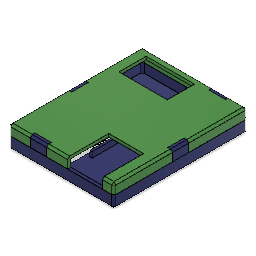
simple-case (Autodesk Fusion 360 design; units mm, degrees)
Autodesk Fusion 360 part; units mm, degrees
sketch "Sketch1" plane through (0, 0, 0) normal (0, 1, 0) x (1, 0, 0) in component "Giraffe"
  line L0 (-22.625, 29.5) -> (22.625, 29.5)
  line L1 (22.625, 29.5) -> (22.625, -29.5)
  line L2 (22.625, -29.5) -> (-22.625, -29.5)
  line L3 (-22.625, -29.5) -> (-22.625, 29.5)
  line L4 (-22.625, 29.5) -> (22.625, -29.5) construction
  line L5 (22.625, 29.5) -> (-22.625, -29.5) construction
  dimension "d1" = 59
  dimension "d2" = 45.25
extrude "Extrude1" add sketch "Sketch1" along normal blind 1.7 makes body 1 in component "Giraffe"
sketch "Sketch2" plane through (0, 0, 0) normal (0, -1, 0) x (1, 0, 0) in component "Giraffe"
  line L0 (22.625, 29.5) -> (-22.625, 29.5)
  line L1 (-22.625, 29.5) -> (-22.625, -29.5)
  line L2 (-22.625, -29.5) -> (22.625, -29.5)
  line L3 (22.625, -29.5) -> (22.625, 29.5)
  line L4 (-3.125, -12) -> (-3.125, 27)
  line L5 (-3.125, 27) -> (-18.125, 23)
  line L6 (-18.125, 23) -> (-18.125, -8)
  line L7 (-18.125, -8) -> (-3.125, -12)
  line L8 (-3.125, 7.5) -> (-13.2165, 7.5) construction
  dimension "d5" = 15
  dimension "d6" = 39
  dimension "d7" = 31
  dimension "d8" = 4.5
  dimension "d9" = 2.5
  measures "d5" distance of L4 L6
  measures "d8" distance of L1 L6
extrude "Extrude2" add sketch "Sketch2" along normal blind 15 separate body contours L4 L5 L6 L7 makes body 2 in component "Giraffe"
fillet "Fillet1" radius 3 4 edges at (-18.125, -7.5, 23) (-3.125, -7.5, 27) (-18.125, -7.5, -8) (-3.125, -7.5, -12) on bodies 2 in component "Giraffe"
sketch "Sketch3" plane through (0, 1.7, 0) normal (0, 1, 0) x (-1, 0, 0) in component "Giraffe"
  line L0 (22.625, 29.5) -> (-22.625, 29.5)
  line L1 (-22.625, 29.5) -> (-22.625, -29.5)
  line L2 (-22.625, -29.5) -> (22.625, -29.5)
  line L3 (22.625, -29.5) -> (22.625, 29.5)
  line L4 (-3.125, 12.5) -> (-20.125, 12.5)
  line L5 (-20.125, 12.5) -> (-20.125, 34.5)
  line L6 (-20.125, 34.5) -> (-3.125, 34.5)
  line L7 (-3.125, 34.5) -> (-3.125, 12.5)
  line L8 (20.325, -29.2) -> (-3.175, -29.2)
  line L9 (-3.175, -29.2) -> (-3.175, -15.95)
  line L10 (-3.175, -15.95) -> (20.325, -15.95)
  line L11 (20.325, -15.95) -> (20.325, -29.2)
  dimension "d13" = 13.25
  dimension "d14" = 23.5
  dimension "d15" = 0.3
  dimension "d16" = 2.3
  dimension "d17" = 17
  dimension "d18" = 22
  dimension "d19" = 2.5
  dimension "d20" = 17
  measures "d14" distance of origin
  measures "d15" distance of L2 L8
  measures "d16" distance of L3 L11
  measures "d18" distance of origin
  measures "d19" distance of L1 L5
  measures "d20" distance of L0 L4
extrude "Extrude4" add sketch "Sketch3" along normal blind 16 separate body contours L8 L9 L10 L11 makes body 3 in component "Giraffe"
extrude "Extrude3" add sketch "Sketch3" along normal blind 14 separate body contours L0 L4 L5 L7 | L0 L5 L6 L7 makes body 4 in component "Giraffe"
sketch "Sketch1 (2)" plane through (0, 1.7, 0) normal (0, 1, 0) x (-1, 0, 0) in component "Top"
  line L0 (22.625, 29.5) -> (-22.625, 29.5)
  line L1 (-22.625, 29.5) -> (-22.625, -29.5)
  line L2 (-22.625, -29.5) -> (22.625, -29.5)
  line L3 (22.625, -29.5) -> (22.625, 29.5)
  line L4 (-25.625, -32.5) -> (25.625, -32.5)
  line L5 (25.625, -32.5) -> (25.625, 32.5)
  line L6 (25.625, 32.5) -> (-25.625, 32.5)
  line L7 (-25.625, 32.5) -> (-25.625, -32.5)
  line L8 (-25.625, -32.5) -> (25.625, 32.5) construction
  line L9 (25.625, -32.5) -> (-25.625, 32.5) construction
  dimension "d25" = 3
  dimension "d26" = 3
  measures "d25" distance of L1 L7
  measures "d26" distance of L2 L4
extrude "Extrude1'" add sketch "Sketch1 (2)" along normal blind 5 separate body contours L0 L1 L2 L3 | L4 L5 L6 L7 makes body 5 in component "Top"
shell "Shell2" thickness 1.5 removed faces 1 at (8.5417, 1.7, 10.8333) on bodies 5 in component "Top"
combine "Combine1" operation cut target body 5 tool bodies 3 4 keep tools in component "Top"
sketch "Sketch2 (2)" plane through (0, 1.7, 0) normal (0, -1, 0) x (1, 0, 0) in component "Base"
  line L0 (3.125, 31) -> (3.125, 32.5)
  line L1 (3.125, 32.5) -> (-25.625, 32.5)
  line L2 (-25.625, 32.5) -> (-25.625, -32.5)
  line L3 (-25.625, -32.5) -> (25.625, -32.5)
  line L4 (25.625, -32.5) -> (25.625, 32.5)
  line L5 (25.625, 32.5) -> (20.125, 32.5)
  line L6 (20.125, 32.5) -> (20.125, 31)
  line L7 (20.125, 31) -> (24.125, 31)
  line L8 (24.125, 31) -> (24.125, -31)
  line L9 (24.125, -31) -> (-24.125, -31)
  line L10 (-24.125, -31) -> (-24.125, 31)
  line L11 (-24.125, 31) -> (3.125, 31)
  line L12 (25.625, -32.5) -> (-25.625, -32.5)
  line L13 (-25.625, -32.5) -> (-25.625, 32.5)
  line L14 (-25.625, 32.5) -> (25.625, 32.5)
  line L15 (25.625, 32.5) -> (25.625, -32.5)
extrude "Extrude1''" add sketch "Sketch2 (2)" along normal blind 6 separate body makes body 6 in component "Base"
shell "Shell1" thickness 1.5 removed faces 1 at (1.0417, 1.7, -10.8333) on bodies 6 in component "Base"
combine "Combine1'" operation cut target body 6 tool bodies 2 keep tools in component "Base"
sketch "Sketch3 (2)" plane through (0, 0, 0) normal (0, 0, 1) x (1, 0, 0) in component "Base"
  line L0 (25.625, 1.7) -> (24.125, 1.7)
  line L1 (24.125, 1.7) -> (24.125, 6.7)
  line L2 (24.125, 6.7) -> (25.625, 6.7)
  line L3 (25.625, 6.7) -> (25.625, 1.7)
  line L4 (25.625, 6.7) -> (-25.625, 6.7)
  line L5 (24.125, 5.2) -> (22.625, 6.7)
  line L6 (23.375, 5.95) -> (23.375, 6.7)
  dimension "d36" = 45
  dimension "d37" = 1.5
  measures "d36" angle of L1 L5
  measures "d37" distance of L4
extrude "Extrude2'" add sketch "Sketch3 (2)" along normal mid plane 8 separate body contours L0 L1 L2 L3 L4 | L1 L4 L5 L6 makes body 7 in component "Base"
chamfer "Chamfer1" distance 1 angle 45 1 edges at (25.625, 6.7, 0) on bodies 7 in component "Base"
mirror "Mirror1" about plane through (0, 0, 0) normal (1, 0, 0) of bodies 7 makes body 8 in component "Base"
copy_body "CopyPasteBodies1" bodies 7 makes body 9 in component "Base"
move_body "Move1" bodies 9 to x (1, 0, 0) y (0, 1, 0) z (0, 0, 1) at (-48.25, 0, 27) in component "Base"
move_body "Move2" bodies 9 to x (0, 0, 1) y (0, 1, 0) z (-1, 0, 0) at (6.875, 0, 55.125) in component "Base"
move_body "Move3" bodies 9 to x (1, 0, 0) y (0, 1, 0) z (0, 0, 1) at (9, 0, 0) in component "Base"
copy_body "CopyPasteBodies2" bodies 7 makes body 10 in component "Base"
move_body "Move4" bodies 10 to x (1, 0, 0) y (0, 1, 0) z (0, 0, 1) at (0, 0, -35) in component "Base"
move_body "Move5" bodies 10 to x (0, 0, -1) y (0, 1, 0) z (1, 0, 0) at (55.125, 0, -6.875) in component "Base"
move_body "Move6" bodies 10 to x (1, 0, 0) y (0, 1, 0) z (0, 0, 1) at (-7, 0, 0) in component "Base"
sketch "Sketch4" plane through (0, -2.8, 0) normal (0, 1, 0) x (-1, 0, 0) in component "Base"
  arc A0 (6.898, 25.9939) -> (3.125, 23.0952) centre (6.125, 23.0952) ccw
  line L0 (6.898, 25.9939) -> (15.898, 23.5939)
  arc A1 (18.125, 20.6952) -> (15.898, 23.5939) centre (15.125, 20.6952) ccw
  line L1 (18.125, 20.6952) -> (18.125, -5.6952)
  arc A2 (15.898, -8.5939) -> (18.125, -5.6952) centre (15.125, -5.6952) ccw
  line L2 (15.898, -8.5939) -> (6.898, -10.9939)
  arc A3 (3.125, -8.0952) -> (6.898, -10.9939) centre (6.125, -8.0952) ccw
  line L3 (3.125, -8.0952) -> (3.125, 23.0952)
  line L4 (24.125, 31) -> (-24.125, 31)
  line L5 (-24.125, 31) -> (-24.125, -31)
  line L6 (-24.125, -31) -> (24.125, -31)
  line L7 (24.125, -31) -> (24.125, 31)
  line L8 (1.125, -17.5) -> (0, -17.5)
  line L9 (0, -17.5) -> (0, 17.5)
  line L10 (0, 17.5) -> (1.125, 17.5)
  line L11 (1.125, 17.5) -> (1.125, -17.5)
  line L12 (0, -0.1553) -> (-18.4041, -0.1553)
  line L13 (-18.4041, -0.1553) -> (-18.4041, 1.3447)
  line L14 (-18.4041, 1.3447) -> (0, 1.3447)
  line L15 (0, 1.3447) -> (0, -0.1553)
  dimension "d42" = 35
  dimension "d43" = 2
  dimension "d44" = 2.125
  dimension "d45" = 1.5
  measures "d43" distance of L3 L11
  measures "d44" distance of L9 L11
  measures "d45" distance of L12 L14
extrude "Extrude3'" add sketch "Sketch4" along normal up to surface (2.8 mm away) contours L8 L9 L10 L11 L15 | L9 L12 L13 L14 L15 bodies 6 in component "Base"
sketch "Sketch2 (3)" plane through (0, 5.2, 0) normal (0, -1, 0) x (1, 0, 0) in component "Top"
  line L0 (3.125, 12.5) -> (3.125, 31)
  line L1 (3.125, 31) -> (-24.125, 31)
  line L2 (-24.125, 31) -> (-24.125, -31)
  line L3 (-24.125, -31) -> (24.125, -31)
  line L4 (24.125, -31) -> (24.125, 31)
  line L5 (24.125, 31) -> (20.125, 31)
  line L6 (20.125, 31) -> (20.125, 12.5)
  line L7 (20.125, 12.5) -> (3.125, 12.5)
  line L8 (-20.325, -29.2) -> (-20.325, -15.95)
  line L9 (-20.325, -15.95) -> (3.175, -15.95)
  line L10 (3.175, -15.95) -> (3.175, -29.2)
  line L11 (3.175, -29.2) -> (-20.325, -29.2)
  line L12 (-1.125, 17.5) -> (0, 17.5)
  line L13 (0, 17.5) -> (0, -17.5)
  line L14 (0, -17.5) -> (-1.125, -17.5)
  line L15 (-1.125, -17.5) -> (-1.125, 17.5)
  line L16 (18.4041, 1.3447) -> (0, 1.3447)
  line L17 (0, 1.3447) -> (0, 0)
  line L18 (0, 0) -> (18.4041, 0)
  line L19 (18.4041, 0) -> (18.4041, 1.3447)
extrude "Extrude2''" add sketch "Sketch2 (3)" along normal up to surface (3.5 mm away) contours L9 L12 L13 L15 L17 | L13 L16 L17 L18 L19 bodies 5 in component "Top"
chamfer "Chamfer1'" distance 1 angle 45 13 edges at (-25.625, 4.2, -32.5) (-25.625, 6.7, 0) (0, 6.7, -32.5) (25.625, 6.7, 0) (22.875, 6.7, 32.5) (-11.25, 6.7, 32.5) (-25.625, 4.2, 32.5) (25.625, 4.2, 32.5) (25.625, 4.2, -32.5) (-24.125, 3.45, 31) (-24.125, 3.45, -31) (24.125, 3.45, 31) (24.125, 3.45, -31) on bodies 5 in component "Top"
chamfer "Chamfer2" distance 1 angle 45 12 edges at (0, -4.3, -32.5) (-25.625, -4.3, 0) (-25.625, -1.3, -32.5) (25.625, -1.3, -32.5) (0, -4.3, 32.5) (-25.625, -1.3, 32.5) (25.625, -1.3, 32.5) (25.625, -4.3, 0) (24.125, -0.55, 31) (24.125, -0.55, -31) (-24.125, -0.55, -31) (-24.125, -0.55, 31) on bodies 6 in component "Base"
combine "Combine2" operation cut target body 5 tool bodies 7 10 8 9 keep tools in component "Top"
component "Giraffe" placed x (1, 0, 0) y (0, 1, 0) z (0, 0, 1) at (0, 0, 0)
component "Base" placed x (1, 0, 0) y (0, 1, 0) z (0, 0, 1) at (0, 0, 0)
component "Top" placed x (1, 0, 0) y (0, 1, 0) z (0, 0, 1) at (0, 0, 0)
equation "d6 = 38 mm + 1 mm"
equation "d7 = 30 mm + 1 mm"
equation "d8 = 5 mm - 0.5 mm"
equation "d9 = 3 mm - 0.5 mm"
equation "d13 = 12.25 mm + 1 mm"
equation "d14 = 22.5 mm + 1 mm"
equation "d15 = 0.8 mm - 0.5 mm"
equation "d16 = 2.8 mm - 0.5 mm"
equation "d17 = 16 mm + 1 mm"
equation "d19 = 3 mm - 0.5 mm"
named bodies: "PCB", "OBD", "RJ-45", "CAN"
